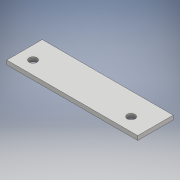
# Autodesk Inventor part: Hinge
Saved by Autodesk Inventor 2018.3 (Build 223284000, 284)
## iProperties
Created: 2018-08-05
Part Number: Hinge
Material: Generic
Document SubType Name: Modeling
Designer: mzhang
Density: 1 g/cm^3
Appearance: Default
Author: mzhang
Autodesk Inventor part; units mm, degrees
ref_plane "YZ Plane" through (0, 0, 0) normal (1, 0, 0) x (0, 1, 0)
ref_plane "XZ Plane" through (0, 0, 0) normal (0, 1, 0) x (-1, 0, 0)
ref_plane "XY Plane" through (0, 0, 0) normal (0, 0, 1) x (1, 0, 0)
sketch "Sketch1" plane through (0, 0, 0) normal (0, 0, 1) x (1, 0, 0)
  line L0 (0, 0) -> (45.0824, 0)
  line L1 (45.0824, 27.0282) -> (0, 27.0282)
  line L2 (0, 27.0282) -> (0, 0)
  circle A0 centre (10, 10) radius 3
  circle A1 centre (84.71, 10) radius 3
  line L3 (99.71, 27.0282) -> (99.71, 0)
  line L4 (45.0824, 27.0282) -> (99.71, 27.0282)
  line L5 (45.0824, 0) -> (99.71, 0)
  dimension "d0" = 6
  dimension "d1" = 10
  dimension "d2" = 10
  dimension "d3" = 6
  dimension "d4" = 74.71
  dimension "d5" = 15
  constraints: 12 end point, 3 horizontal, 2 centre point, 1 parallel, 1 vertical
  measures "d0" diameter of A0
  measures "d1" distance from line of L0 A0.centre
  measures "d2" distance from line of L2 A0.centre
  measures "d3" diameter of A1
  measures "d4" distance of A1.centre A0.centre
  measures "d5" distance from line of L3 A1.centre
extrude "Extrusion1" add sketch "Sketch1" along normal blind 3.175
body "Solid1"
